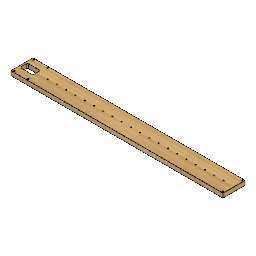
Base plate v38 (Autodesk Fusion 360 design; units mm, degrees)
Autodesk Fusion 360 part; units mm, degrees
sketch "Sketch1" plane through (0, 0, 0) normal (0, 1, 0) x (1, 0, 0)
  line L0 (-300, 30.15) -> (274, 30.15)
  line L1 (274, 30.15) -> (274, -30.15)
  line L2 (274, -30.15) -> (-300, -30.15)
  line L3 (-300, -30.15) -> (-300, 30.15)
  dimension "d1" = 574
  dimension "d2" = 60.3
  dimension "d3" = 300
  dimension "d4" = 30.15
extrude "Extrude1" add sketch "Sketch1" along normal blind 12
sketch "Sketch2" plane through (0, 12, 0) normal (0, 1, 0) x (-1, 0, 0)
  circle A0 centre (256.6, 26.25) radius 2
  line L0 (300, 30.15) -> (-274, 30.15)
  line L1 (300, -30.15) -> (300, 30.15)
  line L2 (256.6, 26.25) -> (294.4, 26.25) construction
  line L3 (294.4, 26.25) -> (294.4, -26.25) construction
  line L4 (294.4, -26.25) -> (256.6, -26.25) construction
  line L5 (256.6, -26.25) -> (256.6, 26.25) construction
  circle A1 centre (294.4, -26.25) radius 2
  circle A2 centre (256.6, -26.25) radius 2
  circle A3 centre (294.4, 26.25) radius 2
  dimension "d9" = 4
  dimension "d13" = 52.5
  dimension "d14" = 37.8
  dimension "d15" = 26.25
  dimension "d16" = 5.6
  dimension "d17" = 4
  dimension "d18" = 4
  dimension "d19" = 4
  measures "d9" diameter of A0
  measures "d17" diameter of A2
  measures "d18" diameter of A1
  measures "d19" diameter of A3
extrude "Extrude2" cut sketch "Sketch2" against normal through all
sketch "Sketch3" plane through (0, 12, 0) normal (0, 1, 0) x (-1, 0, 0)
  circle A0 centre (256.6, 26.25) radius 2
  line L0 (300, 30.15) -> (-274, 30.15)
  line L1 (-274, 30.15) -> (-274, -30.15)
  line L2 (-274, -30.15) -> (300, -30.15)
  line L3 (300, -30.15) -> (300, 30.15)
  circle A1 centre (256.6, -26.25) radius 2
  circle A2 centre (294.4, -26.25) radius 2
  circle A3 centre (294.4, 26.25) radius 2
sketch "Sketch4" plane through (0, 12, 0) normal (0, 1, 0) x (-1, 0, 0)
  line L0 (300, 30.15) -> (-274, 30.15)
  line L1 (-274, 30.15) -> (-274, -30.15)
  line L2 (-274, -30.15) -> (300, -30.15)
  line L3 (300, -30.15) -> (300, 30.15)
  circle A0 centre (256.6, -26.25) radius 2
  circle A1 centre (294.4, -26.25) radius 2
  circle A2 centre (256.6, 26.25) radius 2
  circle A3 centre (294.4, 26.25) radius 2
  circle A4 centre (-270, -26.25) radius 2
  circle A5 centre (-270, 26.25) radius 2
  dimension "d21" = 4
  dimension "d22" = 4
  dimension "d23" = 52.5
  dimension "d26" = 4
  dimension "d27" = 4
  dimension "d30" = 26.25
  measures "d26" diameter of A4
  measures "d27" diameter of A5
extrude "Extrude4" cut sketch "Sketch4" against normal through all contours A4 | A5
sketch "Sketch5" plane through (0, 12, 0) normal (0, 1, 0) x (-1, 0, 0)
  circle A0 centre (-270, -26.25) radius 2
  circle A1 centre (-270, 26.25) radius 2
  line L0 (-274, -30.15) -> (300, -30.15)
  line L1 (300, -30.15) -> (300, 30.15)
  line L2 (300, 30.15) -> (-274, 30.15)
  line L3 (-274, 30.15) -> (-274, -30.15)
  circle A2 centre (256.6, -26.25) radius 2
  circle A3 centre (294.4, -26.25) radius 2
  circle A4 centre (256.6, 26.25) radius 2
  circle A5 centre (294.4, 26.25) radius 2
  line L4 (240, 0) -> (-260, 0) construction
  circle A6 centre (230, 0) radius 1.5
  circle A7 centre (205, 0) radius 1.5
  circle A8 centre (180, 0) radius 1.5
  circle A9 centre (155, 0) radius 1.5
  circle A10 centre (130, 0) radius 1.5
  circle A11 centre (105, 0) radius 1.5
  circle A12 centre (80, 0) radius 1.5
  circle A13 centre (55, 0) radius 1.5
  circle A14 centre (30, 0) radius 1.5
  circle A15 centre (5, 0) radius 1.5
  circle A16 centre (-20, 0) radius 1.5
  circle A17 centre (-45, 0) radius 1.5
  circle A18 centre (-70, 0) radius 1.5
  circle A19 centre (-95, 0) radius 1.5
  circle A20 centre (-120, 0) radius 1.5
  circle A21 centre (-145, 0) radius 1.5
  circle A22 centre (-170, 0) radius 1.5
  circle A23 centre (-195, 0) radius 1.5
  circle A24 centre (-220, 0) radius 1.5
  circle A25 centre (-245, 0) radius 1.5
  dimension "d34" = 60
  dimension "d35" = 10
  dimension "d36" = 3
  dimension "d39" = -25
  dimension "d40" = 0
  dimension "d41" = 500
  dimension "d42" = 25
  dimension "d43" = 15
  measures "d36" diameter of A6
extrude "Extrude5" cut sketch "Sketch5" against normal through all contours A6 | A7 | A8 | A9 | A10 | A11 | A12 | A13 | A14 | A15 | A16 | A17 | A18 | A19 | A20 | A21 | A22 | A23 | A24 | A25
sketch "Sketch6" plane through (0, 0, 0) normal (0, -1, 0) x (1, 0, 0)
  circle A0 centre (195, 0) radius 1.5
  circle A1 centre (95, 0) radius 1.5
  circle A2 centre (-5, 0) radius 1.5
  circle A3 centre (-105, 0) radius 1.5
  circle A4 centre (-205, 0) radius 1.5
  circle A5 centre (-180, 0) radius 1.5
  circle A6 centre (-80, 0) radius 1.5
  circle A7 centre (20, 0) radius 1.5
  circle A8 centre (120, 0) radius 1.5
  circle A9 centre (220, 0) radius 1.5
  circle A10 centre (170, 0) radius 1.5
  circle A11 centre (70, 0) radius 1.5
  circle A12 centre (-30, 0) radius 1.5
  circle A13 centre (-130, 0) radius 1.5
  circle A14 centre (-230, 0) radius 1.5
  circle A15 centre (-155, 0) radius 1.5
  circle A16 centre (-55, 0) radius 1.5
  circle A17 centre (45, 0) radius 1.5
  circle A18 centre (145, 0) radius 1.5
  circle A19 centre (245, 0) radius 1.5
  circle A20 centre (270, -26.25) radius 2
  circle A21 centre (270, 26.25) radius 2
  circle A22 centre (-256.6, -26.25) radius 2
  circle A23 centre (-294.4, -26.25) radius 2
  circle A24 centre (-256.6, 26.25) radius 2
  circle A25 centre (-294.4, 26.25) radius 2
  line L0 (274, -30.15) -> (274, 30.15)
  line L1 (274, 30.15) -> (-300, 30.15)
  line L2 (-300, 30.15) -> (-300, -30.15)
  line L3 (-300, -30.15) -> (274, -30.15)
  line L4 (-292, 10) -> (-263, 10)
  line L5 (-260, 7) -> (-260, -7)
  line L6 (-263, -10) -> (-292, -10)
  line L7 (-295, -7) -> (-295, 7)
  arc A26 (-292, 10) -> (-295, 7) centre (-292, 7) ccw
  arc A27 (-260, 7) -> (-263, 10) centre (-263, 7) ccw
  arc A28 (-263, -10) -> (-260, -7) centre (-263, -7) ccw
  arc A29 (-295, -7) -> (-292, -10) centre (-292, -7) ccw
  dimension "d45" = 20.15
  dimension "d46" = 20
  dimension "d47" = 35
  dimension "d48" = 5
  dimension "d49" = 3
  dimension "d50" = 3
  measures "d45" distance of L1 L4
  measures "d48" distance of L2 L7
  measures "d49" radius of A26
  measures "d50" radius of A29
extrude "Extrude6" cut sketch "Sketch6" against normal through all contours L4 L5 L6 L7 A26 A27 A28 A29
sketch "Sketch8" plane through (0, 0, 0) normal (0, -1, 0) x (1, 0, 0)
  line L0 (-260, 7) -> (-260, -7)
  arc A0 (-263, -10) -> (-260, -7) centre (-263, -7) ccw
  line L1 (-263, -10) -> (-292, -10)
  arc A1 (-295, -7) -> (-292, -10) centre (-292, -7) ccw
  line L2 (-295, -7) -> (-295, 7)
  arc A2 (-292, 10) -> (-295, 7) centre (-292, 7) ccw
  line L3 (-292, 10) -> (-263, 10)
  arc A3 (-260, 7) -> (-263, 10) centre (-263, 7) ccw
  circle A4 centre (195, 0) radius 1.5
  circle A5 centre (95, 0) radius 1.5
  circle A6 centre (-5, 0) radius 1.5
  circle A7 centre (-105, 0) radius 1.5
  circle A8 centre (-205, 0) radius 1.5
  circle A9 centre (-180, 0) radius 1.5
  circle A10 centre (-80, 0) radius 1.5
  circle A11 centre (20, 0) radius 1.5
  circle A12 centre (120, 0) radius 1.5
  circle A13 centre (220, 0) radius 1.5
  circle A14 centre (170, 0) radius 1.5
  circle A15 centre (70, 0) radius 1.5
  circle A16 centre (-30, 0) radius 1.5
  circle A17 centre (-130, 0) radius 1.5
  circle A18 centre (-230, 0) radius 1.5
  circle A19 centre (-155, 0) radius 1.5
  circle A20 centre (-55, 0) radius 1.5
  circle A21 centre (45, 0) radius 1.5
  circle A22 centre (145, 0) radius 1.5
  circle A23 centre (245, 0) radius 1.5
  circle A24 centre (270, -26.25) radius 2
  circle A25 centre (270, 26.25) radius 2
  circle A26 centre (-256.6, -26.25) radius 2
  circle A27 centre (-294.4, -26.25) radius 2
  circle A28 centre (-256.6, 26.25) radius 2
  circle A29 centre (-294.4, 26.25) radius 2
  line L4 (274, -30.15) -> (274, 30.15)
  line L5 (274, 30.15) -> (-300, 30.15)
  line L6 (-300, 30.15) -> (-300, -30.15)
  line L7 (-300, -30.15) -> (274, -30.15)
  circle A30 centre (-230, 0) radius 1.5
  line L8 (-237.5, 3.05) -> (252.5, 3.05)
  line L9 (252.5, 3.05) -> (252.5, -3.05)
  line L10 (252.5, -3.05) -> (-237.5, -3.05)
  line L11 (-237.5, -3.05) -> (-237.5, 3.05)
  line L12 (242.25, 2.75) -> (247.75, 2.75) construction
  line L13 (247.75, 2.75) -> (247.75, -2.75) construction
  line L14 (247.75, -2.75) -> (242.25, -2.75) construction
  line L15 (242.25, -2.75) -> (242.25, 2.75) construction
  circle A31 centre (249.5, 0.05) radius 3 construction
  line L16 (-232.75, 2.75) -> (-227.25, 2.75) construction
  line L17 (-227.25, 2.75) -> (-227.25, -2.75) construction
  line L18 (-227.25, -2.75) -> (-232.75, -2.75) construction
  line L19 (-232.75, -2.75) -> (-232.75, 2.75) construction
  dimension "d54" = 490
  dimension "d55" = 6.1
  dimension "d56" = 3.05
  dimension "d57" = 7.5
  dimension "d64" = 5.5
  dimension "d65" = 5.5
  dimension "d66" = 2.75
  dimension "d67" = 2.75
  dimension "d68" = 6
  dimension "d69" = 90
  dimension "d70" = 90
  dimension "d71" = 90
  dimension "d72" = 90
  dimension "d73" = 5.5
  dimension "d74" = 2.75
  dimension "d75" = 5.5
  dimension "d76" = 2.75
  measures "d56" distance of origin L8
  measures "d57" distance of origin L11
  measures "d66" distance of origin L15
  measures "d67" distance of origin L12
  measures "d68" diameter of A31
  measures "d69" angle of L14 L15
  measures "d70" angle of L13 L14
  measures "d71" angle of L12 L13
  measures "d72" angle of L12 L15
  measures "d74" distance of origin L17
  measures "d76" distance of origin L16
extrude "Extrude7" cut sketch "Sketch8" against normal blind 3 contours L8 L9 L10 L11
extrude "Extrude8" cut 1 faces at (-235.5, 3, 0) along direction (0, 1, 0) blind 3
hole "Hole3" at (251.4393, 0, -1.9893) direction (0, 1, 0) diameter 3 end up to surface (6 mm away)
hole "Hole4" at (-236.4393, 0, -1.9893) direction (0, 1, 0) diameter 3 end up to surface (6 mm away)
hole "Hole5" at (251.4393, 0, 1.9893) direction (0, 1, 0) diameter 3 end up to surface (6 mm away)
hole "Hole6" at (-236.4393, 0, 1.9893) direction (0, 1, 0) diameter 3 end up to surface (6 mm away)
equation "d1 = 600 mm - 19 mm - 7 mm"
equation "d4 = ( 60.3 / 2 ) * 1 mm"
equation "d15 = ( 52.5 / 2 ) * 1 mm"
equation "d34 = 75 mm - 15 mm"
equation "d56 = ( 6.1 / 2 ) * 1 mm"
equation "d66 = ( 5.5 / 2 ) * 1 mm"
equation "d67 = ( 5.5 / 2 ) * 1 mm"
equation "d74 = ( 5.5 / 2 ) * 1 mm"
equation "d76 = ( 5.5 / 2 ) * 1 mm"
equation "dbToolDia = 3 mm"
equation "dbOffset = 0 mm" comment "Do NOT change formula"
equation "dbRadius = ( dbToolDia + dbOffset ) / 2" comment "Do NOT change formula"
equation "dbMinPercent = 10"
equation "dbHoleOffset = dbRadius / sqrt(2)" comment "Do NOT change formula"
equation "d91 = dbRadius * 2"
equation "d93 = dbHoleOffset"
equation "d94 = dbHoleOffset"
equation "d96 = dbRadius * 2"
equation "d98 = dbHoleOffset"
equation "d99 = dbHoleOffset"
equation "d101 = dbRadius * 2"
equation "d103 = dbHoleOffset"
equation "d104 = dbHoleOffset"
equation "d106 = dbRadius * 2"
equation "d108 = dbHoleOffset"
equation "d109 = dbHoleOffset"
